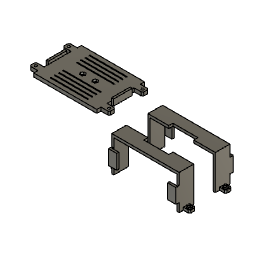
updown_converter_mount (Autodesk Fusion 360 design; units mm, degrees)
Autodesk Fusion 360 part; units mm, degrees
sketch "Sketch1" plane through (0, 0, 0) normal (0, 0, 1) x (1, 0, 0)
  line L0 (0, 0) -> (151.9, 0)
  line L1 (151.9, 0) -> (151.9, -114.75)
  line L2 (151.9, -114.75) -> (0, -114.75)
  line L3 (0, -114.75) -> (0, 0)
  line L4 (0, -10) -> (-5, -10)
  line L5 (-5, -10) -> (-5, -25)
  line L6 (-5, -25) -> (0, -25)
  line L7 (0, -25) -> (0, -10)
  line L8 (-5, -10) -> (-20, -10)
  line L9 (-20, -10) -> (-20, -25)
  line L10 (-20, -25) -> (-5, -25)
  line L11 (-5, -25) -> (-5, -10)
  line L12 (0, -104.75) -> (-5, -104.75)
  line L13 (-5, -104.75) -> (-5, -89.75)
  line L14 (-5, -89.75) -> (0, -89.75)
  line L15 (0, -89.75) -> (0, -104.75)
  line L16 (-5, -89.75) -> (-20, -89.75)
  line L17 (-20, -89.75) -> (-20, -104.75)
  line L18 (-20, -104.75) -> (-5, -104.75)
  line L19 (-5, -104.75) -> (-5, -89.75)
  line L20 (151.9, -10) -> (156.9, -10)
  line L21 (156.9, -10) -> (156.9, -25)
  line L22 (156.9, -25) -> (151.9, -25)
  line L23 (151.9, -25) -> (151.9, -10)
  line L24 (156.9, -10) -> (171.9, -10)
  line L25 (171.9, -10) -> (171.9, -25)
  line L26 (171.9, -25) -> (156.9, -25)
  line L27 (156.9, -25) -> (156.9, -10)
  line L28 (151.9, -104.9495) -> (156.9, -104.9495)
  line L29 (156.9, -104.9495) -> (156.9, -89.9495)
  line L30 (156.9, -89.9495) -> (151.9, -89.9495)
  line L31 (151.9, -89.9495) -> (151.9, -104.9495)
  line L32 (156.9, -89.9495) -> (171.9, -89.9495)
  line L33 (171.9, -89.9495) -> (171.9, -104.9495)
  line L34 (171.9, -104.9495) -> (156.9, -104.9495)
  line L35 (156.9, -104.9495) -> (156.9, -89.9495)
  line L36 (-15.5, -22.6962) -> (-9.5, -22.6962)
  line L37 (-9.5, -22.6962) -> (-6.5, -17.5)
  line L38 (-6.5, -17.5) -> (-9.5, -12.3038)
  line L39 (-9.5, -12.3038) -> (-15.5, -12.3038)
  line L40 (-15.5, -12.3038) -> (-18.5, -17.5)
  line L41 (-18.5, -17.5) -> (-15.5, -22.6962)
  line L42 (-15.5, -22.6962) -> (-9, -22.6962) construction
  circle A0 centre (-12.5, -17.5) radius 3.05
  line L43 (-15.5, -102.4462) -> (-9.5, -102.4462)
  line L44 (-9.5, -102.4462) -> (-6.5, -97.25)
  line L45 (-6.5, -97.25) -> (-9.5, -92.0538)
  line L46 (-9.5, -92.0538) -> (-15.5, -92.0538)
  line L47 (-15.5, -92.0538) -> (-18.5, -97.25)
  line L48 (-18.5, -97.25) -> (-15.5, -102.4462)
  line L49 (-15.5, -102.4462) -> (-16.9999, -102.4462) construction
  circle A1 centre (-12.5, -97.25) radius 3.05
  line L50 (161.4, -22.6962) -> (167.4, -22.6962)
  line L51 (167.4, -22.6962) -> (170.4, -17.5)
  line L52 (170.4, -17.5) -> (167.4, -12.3038)
  line L53 (167.4, -12.3038) -> (161.4, -12.3038)
  line L54 (161.4, -12.3038) -> (158.4, -17.5)
  line L55 (158.4, -17.5) -> (161.4, -22.6962)
  line L56 (161.4, -22.6962) -> (166, -22.6962) construction
  circle A2 centre (164.4, -17.5) radius 3.05
  line L57 (161.4, -102.6456) -> (167.4, -102.6456)
  line L58 (167.4, -102.6456) -> (170.4, -97.4495)
  line L59 (170.4, -97.4495) -> (167.4, -92.2533)
  line L60 (167.4, -92.2533) -> (161.4, -92.2533)
  line L61 (161.4, -92.2533) -> (158.4, -97.4495)
  line L62 (158.4, -97.4495) -> (161.4, -102.6456)
  line L63 (161.4, -102.6456) -> (167.4, -102.6456) construction
  circle A3 centre (164.4, -97.4495) radius 3.05
  line L64 (0, -35) -> (-5, -35)
  line L65 (-5, -35) -> (-5, -79.75)
  line L66 (-5, -79.75) -> (0, -79.75)
  line L67 (0, -79.75) -> (0, -35)
  line L68 (151.9, -35) -> (156.9, -35)
  line L69 (156.9, -35) -> (156.9, -79.75)
  line L70 (156.9, -79.75) -> (151.9, -79.75)
  line L71 (151.9, -79.75) -> (151.9, -35)
  line L72 (25, -57.375) -> (50, -57.375)
  line L73 (50, -57.375) -> (151.9, -57.375)
  line L74 (25, -57.375) -> (0, -57.375)
  line L75 (57.95, -62.5712) -> (63.95, -62.5712)
  line L76 (63.95, -62.5712) -> (66.95, -57.375)
  line L77 (66.95, -57.375) -> (63.95, -52.1788)
  line L78 (63.95, -52.1788) -> (57.95, -52.1788)
  line L79 (57.95, -52.1788) -> (54.95, -57.375)
  line L80 (54.95, -57.375) -> (57.95, -62.5712)
  line L81 (57.95, -62.5712) -> (57.8661, -62.5712) construction
  line L82 (87.95, -62.5712) -> (93.95, -62.5712)
  line L83 (93.95, -62.5712) -> (96.95, -57.375)
  line L84 (96.95, -57.375) -> (93.95, -52.1788)
  line L85 (93.95, -52.1788) -> (87.95, -52.1788)
  line L86 (87.95, -52.1788) -> (84.95, -57.375)
  line L87 (84.95, -57.375) -> (87.95, -62.5712)
  line L88 (87.95, -62.5712) -> (94.0688, -62.5712) construction
  circle A4 centre (60.95, -57.375) radius 3.05
  circle A5 centre (90.95, -57.375) radius 3.05
  line L89 (30, -40) -> (120, -40)
  line L90 (120, -40) -> (120, -42)
  line L91 (120, -42) -> (30, -42)
  line L92 (30, -42) -> (30, -40)
  line L93 (30, -30) -> (120, -30)
  line L94 (120, -30) -> (120, -32)
  line L95 (120, -32) -> (30, -32)
  line L96 (30, -32) -> (30, -30)
  line L97 (30, -20) -> (120, -20)
  line L98 (120, -20) -> (120, -22)
  line L99 (120, -22) -> (30, -22)
  line L100 (30, -22) -> (30, -20)
  line L101 (30, -10) -> (120, -10)
  line L102 (120, -10) -> (120, -12)
  line L103 (120, -12) -> (30, -12)
  line L104 (30, -12) -> (30, -10)
  line L105 (30, -75) -> (120, -75)
  line L106 (120, -75) -> (120, -73)
  line L107 (120, -73) -> (30, -73)
  line L108 (30, -73) -> (30, -75)
  line L109 (30, -85) -> (120, -85)
  line L110 (120, -85) -> (120, -83)
  line L111 (120, -83) -> (30, -83)
  line L112 (30, -83) -> (30, -85)
  line L113 (30, -95) -> (120, -95)
  line L114 (120, -95) -> (120, -93)
  line L115 (120, -93) -> (30, -93)
  line L116 (30, -93) -> (30, -95)
  line L117 (30, -105) -> (120, -105)
  line L118 (120, -105) -> (120, -103)
  line L119 (120, -103) -> (30, -103)
  line L120 (30, -103) -> (30, -105)
  point P0 (-12.5, -17.5)
  point P1 (-12.5, -97.25)
  point P2 (164.4, -17.5)
  point P3 (164.4, -97.4495)
  point P4 (60.95, -57.375)
  point P5 (90.95, -57.375)
  dimension "d1" = 151.9
  dimension "d2" = 114.75
  dimension "d4" = 15
  dimension "d5" = 5
  dimension "d6" = 15
  dimension "d7" = 15
  dimension "d8" = 15
  dimension "d10" = 5
  dimension "d11" = 15
  dimension "d12" = 15
  dimension "d13" = 15
  dimension "d14" = 6
  dimension "d15" = 0
  dimension "d17" = 7.5
  dimension "d18" = 7.5
  dimension "d19" = 6.1
  dimension "d20" = 6
  dimension "d21" = 0
  dimension "d22" = 7.5
  dimension "d23" = 7.5
  dimension "d24" = 6.1
  dimension "d25" = 6
  dimension "d26" = 0
  dimension "d27" = 7.5
  dimension "d28" = 7.5
  dimension "d29" = 6.1
  dimension "d30" = 6
  dimension "d31" = 0
  dimension "d32" = 7.5
  dimension "d33" = 7.5
  dimension "d34" = 6.1
  dimension "d37" = 10
  dimension "d38" = 5
  dimension "d39" = 44.75
  dimension "d40" = 10
  dimension "d42" = 57.375
  dimension "d44" = 6
  dimension "d45" = 0
  dimension "d48" = 6
  dimension "d49" = 0
  dimension "d51" = 6.1
  dimension "d52" = 6.1
  dimension "d53" = 90
  dimension "d54" = 2
  dimension "d55" = 90
  dimension "d56" = 2
  dimension "d57" = 90
  dimension "d58" = 2
  dimension "d59" = 90
  dimension "d60" = 2
  dimension "d61" = 90
  dimension "d62" = 2
  dimension "d63" = 90
  dimension "d64" = 2
  dimension "d65" = 90
  dimension "d66" = 2
  dimension "d67" = 90
  dimension "d68" = 2
  constraint horizontal L0
  constraint vertical L1
  constraint horizontal L2
  constraint vertical L3
  constraint coincident L0.start L3.end
  constraint horizontal L4
  constraint vertical L5
  constraint horizontal L6
  constraint vertical L7
  constraint coincident L3 L4.start
  constraint horizontal L8
  constraint vertical L9
  constraint horizontal L10
  constraint vertical L11
  constraint horizontal L12
  constraint vertical L13
  constraint horizontal L14
  constraint vertical L15
  constraint coincident L3 L12.start
  constraint horizontal L16
  constraint vertical L17
  constraint horizontal L18
  constraint vertical L19
  constraint horizontal L20
  constraint vertical L21
  constraint horizontal L22
  constraint vertical L23
  constraint coincident L1 L20.start
  constraint horizontal L24
  constraint vertical L25
  constraint horizontal L26
  constraint vertical L27
  constraint horizontal L28
  constraint vertical L29
  constraint horizontal L30
  constraint vertical L31
  constraint coincident L1 L28.start
  constraint horizontal L32
  constraint vertical L33
  constraint horizontal L34
  constraint vertical L35
  constraint horizontal L42
  constraint coincident P0 A0.centre
  constraint horizontal L49
  constraint coincident P1 A1.centre
  constraint horizontal L56
  constraint coincident P2 A2.centre
  constraint horizontal L63
  constraint coincident P3 A3.centre
  constraint horizontal L64
  constraint vertical L65
  constraint horizontal L66
  constraint vertical L67
  constraint coincident L3 L64.start
  constraint horizontal L68
  constraint vertical L69
  constraint horizontal L70
  constraint vertical L71
  constraint coincident L1 L68.start
  constraint horizontal L72
  constraint midpoint L71 L73.end
  constraint perpendicular L71 L73
  constraint midpoint L67 L74.end
  constraint perpendicular L67 L74
  constraint horizontal L81
  constraint coincident L73 P4
  constraint horizontal L88
  constraint coincident L73 P5
  constraint coincident P4 A4.centre
  constraint coincident P5 A5.centre
  constraint horizontal L89
  constraint vertical L90
  constraint horizontal L91
  constraint vertical L92
  constraint horizontal L93
  constraint vertical L94
  constraint horizontal L95
  constraint vertical L96
  constraint horizontal L97
  constraint vertical L98
  constraint horizontal L99
  constraint vertical L100
  constraint horizontal L101
  constraint vertical L102
  constraint horizontal L103
  constraint vertical L104
  constraint horizontal L105
  constraint vertical L106
  constraint horizontal L107
  constraint vertical L108
  constraint horizontal L109
  constraint vertical L110
  constraint horizontal L111
  constraint vertical L112
  constraint horizontal L113
  constraint vertical L114
  constraint horizontal L115
  constraint vertical L116
  constraint horizontal L117
  constraint vertical L118
  constraint horizontal L119
  constraint vertical L120
  measures "d1" distance of L0.start L0.end
  measures "d2" distance of L0.start L2.end
  measures "d4" distance of L13.end L12.end
  measures "d5" distance of L20.start L20.end
  measures "d6" distance of L20.start L22.end
  measures "d7" distance of L20.end L24.end
  measures "d8" distance of L20.end L21.end
  measures "d10" distance of L28.start L28.end
  measures "d11" distance of L28.start L30.end
  measures "d12" distance of L29.end L32.end
  measures "d13" distance of L29.end L28.end
  measures "d14" distance of L36.start L36.end
  measures "d15" angle of L36 L42
  measures "d17" distance of L8 P0
  measures "d18" distance of L9 P0
  measures "d19" diameter of A0
  measures "d20" distance of L43.start L43.end
  measures "d21" angle of L43 L49
  measures "d22" distance of L16 P1
  measures "d23" distance of L17 P1
  measures "d24" diameter of A1
  measures "d25" distance of L50.start L50.end
  measures "d26" angle of L50 L56
  measures "d27" distance of L24 P2
  measures "d28" distance of L25 P2
  measures "d29" diameter of A2
  measures "d30" distance of L57.start L57.end
  measures "d31" angle of L57 L63
  measures "d32" distance of L33 P3
  measures "d33" distance of L32 P3
  measures "d34" diameter of A3
  measures "d37" distance of L6 L64
  measures "d38" distance of L68.start L68.end
  measures "d39" distance of L68.start L70.end
  measures "d40" distance of L22 L68
  measures "d42" distance of L0 L72
  measures "d44" distance of L75.start L75.end
  measures "d45" angle of L75 L81
  measures "d48" distance of L82.start L82.end
  measures "d49" angle of L82 L88
  measures "d51" diameter of A4
  measures "d52" diameter of A5
  measures "d53" distance of L89.start L89.end
  measures "d54" distance of L89.start L91.end
  measures "d55" distance of L93.start L93.end
  measures "d56" distance of L93.start L95.end
  measures "d57" distance of L97.start L97.end
  measures "d58" distance of L97.start L99.end
  measures "d59" distance of L101.start L101.end
  measures "d60" distance of L101.start L103.end
  measures "d61" distance of L105.start L105.end
  measures "d62" distance of L105.start L107.end
  measures "d63" distance of L109.start L109.end
  measures "d64" distance of L109.start L111.end
  measures "d65" distance of L113.start L113.end
  measures "d66" distance of L113.start L115.end
  measures "d67" distance of L117.start L117.end
  measures "d68" distance of L117.start L119.end
extrude "Extrude1" add sketch "Sketch1" along normal blind 8.35 contours L0 L1 L3 L7 L23 L67 L71 L72 L73 L74 L77 L78 L79 L84 L85 L86 | L3 L4 L5 L6 L7 L11 | L1 L20 L21 L22 L23 L27 | L5 L8 L9 L10 L11 | L21 L24 L25 L26 L27 | L1 L2 L3 L15 L31 L67 L71 L72 L73 L74 L75 L76 L80 L82 L83 L87 | L3 L12 L13 L14 L15 L19 | L1 L28 L29 L30 L31 L35 | L13 L16 L17 L18 L19 | L29 L32 L33 L34 L35 | L36 L37 L38 L39 L40 L41 | L43 L44 L45 L46 L47 L48 | L50 L51 L52 L53 L54 L55 | L57 L58 L59 L60 L61 L62 makes body 1
extrude "Extrude2" add sketch "Sketch1" along normal blind 3.25 contours L73 L82 L83 L87 A5 | L73 L84 L85 L86 A5 | L73 L77 L78 L79 A4 | L73 L75 L76 L80 A4 bodies 1
extrude "Extrude3" add sketch "Sketch1" along normal blind 15 contours L3 L64 L65 L66 L67 | L1 L68 L69 L70 L71 bodies 1
chamfer "Chamfer1" distance 3 angle 45 8 edges at (-20, -104.75, 4.175) (-20, -89.75, 4.175) (-20, -25, 4.175) (-20, -10, 4.175) (171.9, -10, 4.175) (171.9, -25, 4.175) (171.9, -104.9495, 4.175) (171.9, -89.9495, 4.175) on bodies 1
sketch "Sketch3" plane through (0, 0, 0) normal (0, 0, 1) x (1, 0, 0)
  line L0 (225, -25) -> (376.9, -25)
  line L1 (376.9, -25) -> (376.9, -60)
  line L2 (376.9, -60) -> (225, -60)
  line L3 (225, -60) -> (225, -25)
  line L4 (270, -60) -> (330, -60)
  line L5 (330, -60) -> (330, -50)
  line L6 (330, -50) -> (270, -50)
  line L7 (270, -50) -> (270, -60)
  line L8 (225, -25) -> (220, -25)
  line L9 (220, -25) -> (220, -60)
  line L10 (220, -60) -> (225, -60)
  line L11 (225, -60) -> (225, -25)
  line L12 (376.9, -25) -> (381.9, -25)
  line L13 (381.9, -25) -> (381.9, -60)
  line L14 (381.9, -60) -> (376.9, -60)
  line L15 (376.9, -60) -> (376.9, -25)
  dimension "d76" = 151.9
  dimension "d78" = 5
  dimension "d79" = 35
  dimension "d80" = 5
  dimension "d81" = 35
  constraint horizontal L0
  constraint vertical L1
  constraint horizontal L2
  constraint vertical L3
  constraint horizontal L4
  constraint vertical L5
  constraint horizontal L6
  constraint vertical L7
  constraint coincident L2 L4.start
  constraint horizontal L8
  constraint vertical L9
  constraint horizontal L10
  constraint vertical L11
  constraint horizontal L12
  constraint vertical L13
  constraint horizontal L14
  constraint vertical L15
  measures "d76" distance of L0.start L0.end
  measures "d78" distance of L0.start L8.end
  measures "d79" distance of L0.start L2.end
  measures "d80" distance of L0.end L12.end
  measures "d81" distance of L0.end L1.end
extrude "Extrude4" add sketch "Sketch3" along normal blind 6.35 separate body contours L0 L1 L2 L3 L5 L6 L7 L11 L15 | L3 L8 L9 L10 L11 | L1 L12 L13 L14 L15 makes body 2
extrude "Extrude5" add sketch "Sketch3" against normal blind 77.25 contours L3 L8 L9 L10 L11 | L1 L12 L13 L14 L15 bodies 2
sketch "Sketch4" plane through (381.9, 0, 0) normal (1, 0, 0) x (0, 1, 0)
  line L0 (-25, -77.25) -> (-25, 6.35)
  line L1 (-25, 6.35) -> (-60, 6.35)
  line L2 (-60, 6.35) -> (-60, -77.25)
  line L3 (-60, -77.25) -> (-25, -77.25)
  line L4 (-60, -77.25) -> (-25, -77.25)
  line L5 (-25, -77.25) -> (-25, -70.9)
  line L6 (-25, -70.9) -> (-60, -70.9)
  line L7 (-60, -70.9) -> (-60, -77.25)
  line L8 (-50, -77.25) -> (-35, -77.25)
  line L9 (-35, -77.25) -> (-35, -70.9)
  line L10 (-35, -70.9) -> (-50, -70.9)
  line L11 (-50, -70.9) -> (-50, -77.25)
  dimension "d86" = 6.35
  dimension "d87" = 15
  dimension "d88" = 10
  constraint horizontal L4
  constraint vertical L5
  constraint horizontal L6
  constraint vertical L7
  constraint coincident L0 L5.end
  constraint coincident L2.end L3.start
  constraint horizontal L8
  constraint vertical L9
  constraint horizontal L10
  constraint vertical L11
  constraint coincident L3 L8.start
  measures "d86" distance of L2.end L6.end
  measures "d87" distance of L8.start L8.end
  measures "d88" distance of L7 L11
extrude "Extrude6" add sketch "Sketch4" along normal blind 15 contours L3 L4 L6 L8 L9 L10 L11 bodies 2
sketch "Sketch5" plane through (0, 0, -70.9) normal (0, 0, 1) x (-1, 0, 0)
  line L0 (-381.9, 35) -> (-381.9, 50)
  line L1 (-381.9, 50) -> (-396.9, 50)
  line L2 (-396.9, 50) -> (-396.9, 35)
  line L3 (-396.9, 35) -> (-381.9, 35)
  line L4 (-386.4, 47.6962) -> (-392.4, 47.6962)
  line L5 (-392.4, 47.6962) -> (-395.4, 42.5)
  line L6 (-395.4, 42.5) -> (-392.4, 37.3038)
  line L7 (-392.4, 37.3038) -> (-386.4, 37.3038)
  line L8 (-386.4, 37.3038) -> (-383.4, 42.5)
  line L9 (-383.4, 42.5) -> (-386.4, 47.6962)
  line L10 (-386.4, 47.6962) -> (-380.4, 47.6962) construction
  circle A0 centre (-389.4, 42.5) radius 3.05
  point P0 (-389.4, 42.5)
  dimension "d91" = 6
  dimension "d93" = 7.5
  dimension "d94" = 7.5
  dimension "d95" = 6.1
  constraint horizontal L10
  constraint coincident P0 A0.centre
  measures "d91" distance of L4.start L4.end
  measures "d93" distance of L1 P0
  measures "d94" distance of L2 P0
  measures "d95" diameter of A0
extrude "Extrude7" cut sketch "Sketch5" against normal blind 6.35 contours A0 bodies 2
extrude "Extrude8" cut sketch "Sketch5" against normal blind 3 contours L4 L5 L6 L7 L8 L9 bodies 2
sketch "Sketch6" plane through (220, 0, 0) normal (-1, 0, 0) x (0, -1, 0)
  line L0 (60, -77.25) -> (60, 6.35)
  line L1 (60, 6.35) -> (25, 6.35)
  line L2 (25, 6.35) -> (25, -77.25)
  line L3 (25, -77.25) -> (60, -77.25)
  line L4 (35, -77.25) -> (50, -77.25)
  line L5 (50, -77.25) -> (50, -70.9)
  line L6 (50, -70.9) -> (35, -70.9)
  line L7 (35, -70.9) -> (35, -77.25)
  dimension "d100" = 15
  dimension "d101" = 6.35
  dimension "d102" = 10
  constraint horizontal L4
  constraint vertical L5
  constraint horizontal L6
  constraint vertical L7
  constraint coincident L3 L4.start
  measures "d100" distance of L4.start L4.end
  measures "d101" distance of L4.start L6.end
  measures "d102" distance of L0 L5
extrude "Extrude9" add sketch "Sketch6" along normal blind 15 contours L3 L4 L5 L6 L7 bodies 2
sketch "Sketch7" plane through (0, 0, -70.9) normal (0, 0, 1) x (-1, 0, 0)
  line L0 (-220, 50) -> (-220, 35)
  line L1 (-220, 35) -> (-205, 35)
  line L2 (-205, 35) -> (-205, 50)
  line L3 (-205, 50) -> (-220, 50)
  line L4 (-209.5, 47.6962) -> (-215.5, 47.6962)
  line L5 (-215.5, 47.6962) -> (-218.5, 42.5)
  line L6 (-218.5, 42.5) -> (-215.5, 37.3038)
  line L7 (-215.5, 37.3038) -> (-209.5, 37.3038)
  line L8 (-209.5, 37.3038) -> (-206.5, 42.5)
  line L9 (-206.5, 42.5) -> (-209.5, 47.6962)
  circle A0 centre (-212.5, 42.5) radius 3.05
  point P0 (-212.5, 42.5)
  dimension "d105" = 6
  dimension "d107" = 7.5
  dimension "d108" = 7.5
  dimension "d109" = 6.1
  constraint coincident P0 A0.centre
  measures "d105" distance of L4.start L4.end
  measures "d107" distance of L3 P0
  measures "d108" distance of L2 P0
  measures "d109" diameter of A0
extrude "Extrude10" cut sketch "Sketch7" against normal blind 6.35 contours A0 bodies 2
extrude "Extrude11" cut sketch "Sketch7" against normal blind 3 contours L4 L5 L6 L7 L8 L9 bodies 2
sketch "Sketch8" plane through (0, -25, 0) normal (0, 1, 0) x (-1, 0, 0)
  line L0 (-220, -77.25) -> (-220, 6.35)
  line L1 (-220, 6.35) -> (-381.9, 6.35)
  line L2 (-381.9, 6.35) -> (-381.9, -77.25)
  line L3 (-381.9, -77.25) -> (-376.9, -77.25)
  line L4 (-376.9, -77.25) -> (-376.9, 0)
  line L5 (-376.9, 0) -> (-225, 0)
  line L6 (-225, 0) -> (-225, -77.25)
  line L7 (-225, -77.25) -> (-220, -77.25)
  line L8 (-381.9, -21.125) -> (-376.9, -21.125)
  line L9 (-376.9, -21.125) -> (-376.9, -56.125)
  line L10 (-376.9, -56.125) -> (-381.9, -56.125)
  line L11 (-381.9, -56.125) -> (-381.9, -21.125)
  line L12 (-225, -56.125) -> (-220, -56.125)
  line L13 (-220, -56.125) -> (-220, -21.125)
  line L14 (-220, -21.125) -> (-225, -21.125)
  line L15 (-225, -21.125) -> (-225, -56.125)
  dimension "d114" = 35
  dimension "d115" = 21.125
  dimension "d116" = 35
  dimension "d117" = 21.125
  constraint horizontal L8
  constraint vertical L9
  constraint horizontal L10
  constraint vertical L11
  constraint coincident L2 L8.start
  constraint horizontal L12
  constraint vertical L13
  constraint horizontal L14
  constraint vertical L15
  constraint coincident L6 L12.start
  measures "d114" distance of L8.start L10.end
  measures "d115" distance of L3 L10
  measures "d116" distance of L12.start L14.end
  measures "d117" distance of L7 L12
extrude "Extrude12" add sketch "Sketch8" along normal blind 8 contours L0 L6 L12 L13 L14 L15 | L2 L4 L8 L9 L10 L11 bodies 2
sketch "Sketch9" plane through (376.9, 0, 0) normal (-1, 0, 0) x (0, -1, 0)
  line L0 (60, 0) -> (25, 0)
  line L1 (25, 0) -> (25, -21.125)
  line L2 (25, -21.125) -> (17, -21.125)
  line L3 (17, -21.125) -> (17, -56.125)
  line L4 (17, -56.125) -> (25, -56.125)
  line L5 (25, -56.125) -> (25, -77.25)
  line L6 (25, -77.25) -> (60, -77.25)
  line L7 (60, -77.25) -> (60, 0)
  line L8 (17, -21.125) -> (22, -21.125)
  line L9 (22, -21.125) -> (22, -56.125)
  line L10 (22, -56.125) -> (17, -56.125)
  line L11 (17, -56.125) -> (17, -21.125)
  line L12 (22, -21.125) -> (25, -21.125)
  line L13 (25, -21.125) -> (25, -56.125)
  line L14 (25, -56.125) -> (22, -56.125)
  line L15 (22, -56.125) -> (22, -21.125)
  dimension "d120" = 5
  constraint horizontal L8
  constraint vertical L9
  constraint horizontal L10
  constraint vertical L11
  constraint coincident L2.end L3.start
  constraint horizontal L12
  constraint vertical L13
  constraint horizontal L14
  constraint vertical L15
  constraint coincident L4.end L5.start
  measures "d120" distance of L2.end L8.end
extrude "Extrude13" add sketch "Sketch9" along normal blind 15 contours L2 L3 L4 L8 L9 L10 L11 L15 bodies 2
extrude "Extrude14" cut sketch "Sketch9" against normal blind 2 contours L2 L4 L9 L12 L13 L14 L15 bodies 2
sketch "Sketch10" plane through (225, 0, 0) normal (1, 0, 0) x (0, 1, 0)
  line L0 (-25, 0) -> (-60, 0)
  line L1 (-60, 0) -> (-60, -77.25)
  line L2 (-60, -77.25) -> (-25, -77.25)
  line L3 (-25, -77.25) -> (-25, -56.125)
  line L4 (-25, -56.125) -> (-17, -56.125)
  line L5 (-17, -56.125) -> (-17, -21.125)
  line L6 (-17, -21.125) -> (-25, -21.125)
  line L7 (-25, -21.125) -> (-25, 0)
  line L8 (-17, -21.125) -> (-22, -21.125)
  line L9 (-22, -21.125) -> (-22, -56.125)
  line L10 (-22, -56.125) -> (-17, -56.125)
  line L11 (-17, -56.125) -> (-17, -21.125)
  line L12 (-25, -21.125) -> (-22, -21.125)
  line L13 (-22, -21.125) -> (-22, -56.125)
  line L14 (-22, -56.125) -> (-25, -56.125)
  line L15 (-25, -56.125) -> (-25, -21.125)
  dimension "d125" = 5
  constraint horizontal L8
  constraint vertical L9
  constraint horizontal L10
  constraint vertical L11
  constraint coincident L5.end L6.start
  constraint horizontal L12
  constraint vertical L13
  constraint horizontal L14
  constraint vertical L15
  constraint coincident L6.end L7.start
  measures "d125" distance of L5.end L8.end
extrude "Extrude15" add sketch "Sketch10" along normal blind 15 contours L4 L5 L6 L8 L9 L10 L11 L13 bodies 2
extrude "Extrude16" cut sketch "Sketch10" against normal blind 2 contours L4 L6 L9 L12 L13 L14 L15 bodies 2
chamfer "Chamfer2" distance 3 angle 45 4 edges at (205, -35, -74.075) (205, -50, -74.075) (396.9, -50, -74.075) (396.9, -35, -74.075) on bodies 2
copy_body "CopyPasteBodies1" bodies 2 makes body 3
move_body "Move1" bodies 3 to x (-1, 0, 0) y (0, -1, 0) z (0, 0, 1) at (600, -170, 0)
equation "d118 = 5 mm + 2.5 mm + 0.5 mm"
